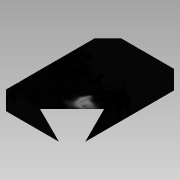
# Autodesk Inventor part: 02_Akku
Saved by Autodesk Inventor 2015 (Build 190159000, 159)
## iProperties
Created: 2015-10-13
Part Number: 02_Akku
Material: Generisch
Document SubType Name: Modeling
Designer: Bene
Density: 1 g/cm^3
Appearance: Schwarz
Author: Bene
Autodesk Inventor part; units mm, degrees
ref_plane "YZ Plane" through (0, 0, 0) normal (1, 0, 0) x (0, 1, 0)
ref_plane "XZ Plane" through (0, 0, 0) normal (0, 1, 0) x (-1, 0, 0)
ref_plane "XY Plane" through (0, 0, 0) normal (0, 0, 1) x (1, 0, 0)
sketch "Skizze1" plane through (0, 0, 0) normal (0, 0, 1) x (1, 0, 0)
  line L0 (-23, -28) -> (23, -28) projected
  line L1 (23, -28) -> (23, -18.5) projected
  line L2 (23, -18.5) -> (12.0668, -18.5) projected
  line L3 (12.0668, -18.5) -> (12.0668, -10.5) projected
  line L4 (12.0668, -10.5) -> (23, -10.5) projected
  line L5 (23, -10.5) -> (23, 33.5) projected
  line L6 (-23, 33.5) -> (-23, -13.75) projected
  line L7 (-23, -13.75) -> (-11.9215, -13.75) projected
  line L8 (-11.9215, -13.75) -> (-11.9215, -19.25) projected
  line L9 (-11.9215, -19.25) -> (-23, -19.25) projected
  line L10 (-23, -19.25) -> (-23, -28) projected
  line L11 (17.5, -28) -> (-17.5, -28)
  line L12 (-17.5, -28) -> (-17.5, 26)
  line L13 (-17.5, 26) -> (17.5, 26)
  line L14 (17.5, 26) -> (17.5, -28)
  line L15 (1.2993, 33.5) -> (1.2993, 28.5) projected
  line L16 (1.2993, 28.5) -> (-14.2007, 28.5) projected
  line L17 (-14.2007, 28.5) -> (-14.2007, 33.5) projected
  line L18 (-14.2007, 33.5) -> (-23, 33.5) projected
  line L19 (23, 33.5) -> (1.2993, 33.5) projected
  circle A0 centre (-20, 29) radius 1 projected
  circle A1 centre (20, 29) radius 1 projected
  point P0 (0, 0)
  dimension "d0" = 54
  dimension "d1" = 5.5
  dimension "d2" = 5.5
  constraints: 8 end point, 2 parallel, 1 horizontal, 1 perpendicular, 1 point on line
  measures "d0" distance of L11.end L12.end
  measures "d1" distance between parallel lines of L14 L5
  measures "d2" distance between parallel lines of L6 L12
extrude "Extrusion1" add sketch "Skizze1" along normal blind 10 contours L12 L9 L8 L7 L13 L14 L4 L3 L2 L0 | L12 L7 L8 L9 | L2 L3 L4 L14
